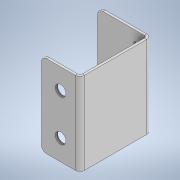
# Autodesk Inventor part: Soporte final de carrera
Saved by Autodesk Inventor 2021 (Build 250183000, 183)
## iProperties
Created: 2021-06-22
Part Number: Soporte final de carrera
Material: Generic
Document SubType Name: Sheet Metal
Designer: Nelson
Density: 1 g/cm^3
Sheet Metal Rule: Default_mm
Appearance: Default
Author: Nelson
Autodesk Inventor part; units mm, degrees
ref_plane "YZ Plane" through (0, 0, 0) normal (1, 0, 0) x (0, 1, 0)
ref_plane "XZ Plane" through (0, 0, 0) normal (0, 1, 0) x (-1, 0, 0)
ref_plane "XY Plane" through (0, 0, 0) normal (0, 0, 1) x (1, 0, 0)
sketch "Sketch2" plane through (0, 0, 0) normal (0, 0, 1) x (1, 0, 0)
  line L0 (0, 0) -> (20, 0)
  line L1 (20, 0) -> (20, 32)
  line L2 (20, 32) -> (0, 32)
  line L3 (0, 32) -> (0, 0)
  dimension "d0" = 20
  dimension "d1" = 32
  measures "d0" distance of L2.end L1.end
  measures "d1" distance of L1.end L0.end
extrude "Plate1" add sketch "Sketch2" along normal blind 0.92
sketch "Sketch3" plane through (19.08, 32, 0) normal (1, 0, 0) x (0, 1, 0)
  line L0 (-32, 0) -> (0, 0)
  line L1 (0, 0) -> (0, 27.8)
  line L2 (0, 27.8) -> (-32, 27.8)
  line L3 (-32, 27.8) -> (-32, 0)
  constraints: 6 end point, 1 horizontal, 1 perpendicular, 1 vertical
edge flange "Flange1" height 27.8 angle 90 thickness 0.92 bend radius 0.92 thickness toward (1, 0, 0) relief straight relief width 0.92 relief depth 0.46 edges at (20, 16, 0.92) wall of the first edge with corners at (19.08, 0, 0) (19.08, 32, 0) (19.08, 32, 27.8) (19.08, 0, 27.8)
bend "Bend1"
corner "Corner1"
sketch "Sketch4" plane through (20, 32, 26.88) normal (0, 0, 1) x (1, 0, 0)
  line L0 (0, -32) -> (0, 0)
  line L1 (0, 0) -> (-15, 0)
  line L2 (-15, 0) -> (-15, -32)
  line L3 (-15, -32) -> (0, -32)
  constraints: 6 end point, 1 horizontal, 1 perpendicular, 1 vertical
edge flange "Flange2" height 15 angle 90 thickness 0.92 bend radius 0.92 thickness toward (0, 0, 1) relief straight relief width 0.92 relief depth 0.46 edges at (19.08, 16, 27.8) wall of the first edge with corners at (20, 0, 26.88) (20, 32, 26.88) (5, 32, 26.88) (5, 0, 26.88)
bend "Bend2"
corner "Corner2"
fillet "Fillet2" radius 2 4 edges at (0, 0, 0.46) (5, 0, 27.34) (5, 32, 27.34) (0, 32, 0.46)
sketch "Sketch5" plane through (0, 0, 0) normal (0, 0, -1) x (-1, 0, 0)
  line L0 (-20, 0) -> (-20, 32) projected
  line L1 (-18.16, 32) -> (-2, 32) projected
  line L2 (0, 30) -> (0, 2) projected
  line L3 (-2, 0) -> (-18.16, 0) projected
  point P0 (0, 0)
  point P1 (-15.15, 27.1)
  point P2 (-4.85, 4.9)
  dimension "d35" = 4.85
  dimension "d36" = 4.9
  dimension "d37" = 4.9
  dimension "d38" = 4.85
  measures "d35" distance from line of L2 point (-4.85, 4.9)
  measures "d36" distance from line of L3 point (-4.85, 4.9)
  measures "d37" distance from line of L1 point (-15.15, 27.1)
  measures "d38" distance from line of point (-15.15, 27.1) L0
hole "Hole1" at (15.15, 27.1, 0) at (4.85, 4.9, 0) direction (0, 0, 1) diameter 2.459 depth 2 tip angle 137 thread size "M3x0.5" class "6H" standard "ISO Metric profile"
sketch "Sketch6" plane through (18.16, 0, 27.8) normal (0, 0, 1) x (1, 0, 0)
  line L0 (-11.16, 32) -> (0, 32) projected
  line L1 (0, 0) -> (-11.16, 0) projected
  line L2 (-13.16, 2) -> (-13.16, 30) projected
  point P0 (-18.16, 0)
  point P1 (-5.66, 24)
  point P2 (-5.66, 8)
  dimension "d46" = 8
  dimension "d47" = 8
  dimension "d48" = 7.5
  dimension "d49" = 7.5
  measures "d46" distance from line of L0 point (-5.66, 24)
  measures "d47" distance from line of L1 point (-5.66, 8)
  measures "d48" distance from line of L2 point (-5.66, 8)
  measures "d49" distance from line of L2 point (-5.66, 24)
hole "Hole2" at (12.5, 24, 27.8) at (12.5, 8, 27.8) direction (0, 0, -1) diameter 4.134 depth 2 tip angle 137 thread size "M5x0.8" class "6H" standard "ISO Metric profile"
equation "\"d2\" = Thickness"
equation "\"d3\" = BendReliefWidth"
equation "\"d4\" = BendReliefDepth"
equation "\"d5\" = MinimumRemnant"
equation "\"d6\" = TransitionRadius"
equation "\"d9\" = BendRadius"
equation "\"d10\" = CornerReliefSize"
equation "\"d11\" = GapSize"
equation "\"d12\" = JacobiRadiusSize"
equation "\"GapSize\" = Thickness"
equation "\"BendRadius\" = Thickness"
equation "\"MinimumRemnant\" = 2 * Thickness"
equation "\"BendReliefDepth\" = 0.5 * Thickness"
equation "\"BendReliefWidth\" = Thickness"
equation "\"CornerReliefSize\" = 4 * Thickness"
equation "\"JacobiRadiusSize\" = BendRadius"
equation "\"TransitionRadius\" = BendRadius"
equation "\"d13\" = BendReliefWidth"
equation "\"d14\" = BendReliefDepth"
equation "\"d15\" = MinimumRemnant"
equation "\"d16\" = TransitionRadius"
equation "\"d19\" = BendRadius"
equation "\"d20\" = CornerReliefSize"
equation "\"d21\" = GapSize"
equation "\"d22\" = JacobiRadiusSize"
equation "\"Thickness\" = 0.92"
body "Solid1"
